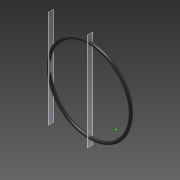
# Autodesk Inventor part: Dętka_koła_tylnego
Saved by Autodesk Inventor 2015 (Build 190159000, 159)
## iProperties
Created: 2015-12-01
Part Number: Dętka_koła_tylnego
Material: Kauczuk
Document SubType Name: Modeling
Designer: graaapsik
Density: 0.93 g/cm^3
Appearance: Kauczuk - czarny - wersja 1.1
Mass: 110.725 g
Surface Area: 2645.52 cm^2
Volume: 119.059 cm^3
Author: graaapsik
Autodesk Inventor part; units mm, degrees
ref_plane "YZ Plane" through (0, 0, 0) normal (1, 0, 0) x (0, 1, 0)
ref_plane "XZ Plane" through (0, 0, 0) normal (0, 1, 0) x (-1, 0, 0)
ref_plane "XY Plane" through (0, 0, 0) normal (0, 0, 1) x (1, 0, 0)
sketch "Szkic1" plane through (0, 0, 0) normal (1, 0, 0) x (0, 1, 0)
  circle A0 centre (0, 303.3215) radius 11.5
  line L0 (0, 0) -> (60.5344, 0) construction
  line L1 (0, 0) -> (0, 55.1671) construction
  line L2 (-16.0424, 302.375) -> (-13.9679, 299.9026) construction
  line L3 (13.9679, 299.9026) -> (16.0424, 302.375) construction
  circle A1 centre (0, 303.3215) radius 10.6
  arc A2 (-6.9613, 292.3237) -> (6.9613, 292.3237) centre (0, 340.3215) ccw construction
  dimension "d0" = 23
  dimension "d1" = 0.9
  constraints: 8 end point, 3 centre point, 2 point on circle, 1 horizontal, 1 perpendicular, 1 point on line, 1 tangent, 8 other
  measures "d0" diameter of A0
  measures "d1" radial gap between concentric circles of A0 A1
revolve "Obrót1" add sketch "Szkic1" angle 360 about axis through (0, 0, 0) along (0, 1, 0)
ref_plane "Płaszczyzna do otworu na wentyl 1" through (0, 0, 0) normal (1, 0, 0) x (0, -1, 0)
ref_plane "Płaszczyzna do otworu na wentyl 1.1" through (-290, 0, 0) normal (1, 0, 0) x (0, -1, 0)
sketch "Szkic4" plane through (-290, 0, 0) normal (1, 0, 0) x (0, -1, 0)
  point P0 (0, 0)
  point P1 (0, 0)
  constraints: 1 coincident
hole "Otwór na wentyl" at (-290, 0, 0) direction (-1, 0, 0) diameter 8.3 depth 8 tip angle 118
